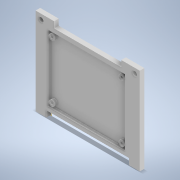
# Autodesk Inventor part: RelayTray
Saved by Autodesk Inventor 2022 (Build 260153000, 153)
## iProperties
Created: 2022-01-15
Part Number: RelayTray
Material: Generic
Document SubType Name: Modeling
Designer: siwat
Density: 1 g/cm^3
Appearance: Default
VLDS_Profile: Default Part
VLDS_TimeStamp: 2022-02-27
VLDS_FailCnt: 3
VLDS_AcceptCnt: 0
Author: siwat
Autodesk Inventor part; units mm, degrees
ref_plane "YZ Plane" through (0, 0, 0) normal (1, 0, 0) x (0, 1, 0)
ref_plane "XZ Plane" through (0, 0, 0) normal (0, 1, 0) x (-1, 0, 0)
ref_plane "XY Plane" through (0, 0, 0) normal (0, 0, 1) x (1, 0, 0)
ref_plane "Work Plane1" through (-62.4151, 1.9295, 0) normal (0, 0, 1) x (1, 0, 0)
sketch "Sketch1" plane through (-62.4151, 1.9295, 0) normal (0, 0, 1) x (1, 0, 0)
  line L0 (-5.0959, -1.798) -> (62.2123, -1.798)
  line L1 (62.2123, -1.798) -> (62.2123, 54.509)
  line L2 (62.2123, 54.509) -> (-5.0959, 54.509)
  line L3 (-5.0959, 54.509) -> (-5.0959, -1.798)
  circle A0 centre (-1.5532, 51.0932) radius 1.5
  circle A1 centre (58.9247, 51.1571) radius 1.5
  point P0 (62.4151, -1.9295)
  dimension "d1" = 3
  dimension "d6" = 3
  constraints: 8 end point, 2 centre point, 2 parallel, 1 horizontal, 1 perpendicular
  measures "d1" diameter of A0
  measures "d6" diameter of A1
extrude "Extrusion1" add sketch "Sketch1" along normal blind 3
sketch "Sketch3" plane through (-62.4151, 1.9295, 3) normal (0, 0, 1) x (1, 0, 0)
  line L0 (52.7586, 47.7976) -> (2.7586, 47.7976)
  line L1 (2.7586, 47.7976) -> (2.7586, 4.7976)
  line L2 (2.7586, 4.7976) -> (52.7586, 4.7976)
  line L3 (52.7586, 4.7976) -> (52.7586, 47.7976)
  circle A0 centre (5.2586, 7.7976) radius 1
  circle A1 centre (5.2586, 7.7976) radius 1.85
  circle A2 centre (50.2586, 7.7976) radius 1
  circle A3 centre (50.2586, 7.7976) radius 1.85
  circle A4 centre (50.2586, 44.7976) radius 1
  circle A5 centre (50.2586, 44.7976) radius 1.85
  circle A6 centre (5.2586, 44.7976) radius 1
  circle A7 centre (5.2586, 44.7976) radius 1.85
  point P0 (62.4151, -1.9295)
  dimension "d7" = 50
  dimension "d8" = 43
  dimension "d9" = 2
  dimension "d10" = 3.7
  dimension "d11" = 3
  dimension "d12" = 2.5
  dimension "d13" = 2
  dimension "d14" = 3.7
  dimension "d15" = 2
  dimension "d16" = 3.7
  dimension "d17" = 2
  dimension "d18" = 3.7
  dimension "d19" = 3
  dimension "d20" = 2.5
  dimension "d21" = 2.5
  dimension "d22" = 3
  dimension "d23" = 2.5
  dimension "d24" = 3
  constraints: 8 centre point, 8 end point, 4 coincident, 2 parallel, 1 horizontal, 1 perpendicular
  measures "d7" distance of L1.end L2.end
  measures "d8" distance of L2.end L0.start
  measures "d9" diameter of A0
  measures "d10" diameter of A1
  measures "d11" distance from line of A0.centre L2
  measures "d12" distance from line of L1 A0.centre
  measures "d13" diameter of A2
  measures "d14" diameter of A3
  measures "d15" diameter of A4
  measures "d16" diameter of A5
  measures "d17" diameter of A6
  measures "d18" diameter of A7
  measures "d19" distance from line of L0 A6.centre
  measures "d20" distance from line of L1 A6.centre
  measures "d21" distance from line of L3 A4.centre
  measures "d22" distance from line of L0 A4.centre
  measures "d23" distance from line of L3 A2.centre
  measures "d24" distance from line of A2.centre L2
extrude "Extrusion3" cut sketch "Sketch3" against normal blind 2
sketch "Sketch4" plane through (-62.4151, 1.9295, 1) normal (0, 0, 1) x (1, 0, 0)
  circle A0 centre (50.2586, 7.7976) radius 1 projected
  circle A1 centre (50.2586, 7.7976) radius 1
  circle A2 centre (50.2586, 44.7976) radius 1 projected
  circle A3 centre (50.2586, 44.7976) radius 1
  circle A4 centre (5.2586, 44.7976) radius 1 projected
  circle A5 centre (5.2586, 44.7976) radius 1
  circle A6 centre (5.2586, 7.7976) radius 1 projected
  circle A7 centre (5.2586, 7.7976) radius 1
  point P0 (62.4151, -1.9295)
  constraints: 4 centre point, 4 coincident
extrude "Extrusion4" cut sketch "Sketch4" against normal through all
sketch "Sketch5" plane through (-62.4151, 1.9295, 3) normal (0, 0, 1) x (1, 0, 0)
  line L0 (-5.0959, -1.798) -> (62.2123, -1.798) projected
  line L1 (55.2123, -1.798) -> (1.9041, -1.798)
  line L2 (1.9041, -1.798) -> (1.9041, 2.202)
  line L3 (1.9041, 2.202) -> (55.2123, 2.202)
  line L4 (55.2123, 2.202) -> (55.2123, -1.798)
  line L5 (62.2123, 54.509) -> (-5.0959, 54.509) projected
  line L6 (6.9041, 54.509) -> (50.2123, 54.509)
  line L7 (50.2123, 54.509) -> (50.2123, 50.509)
  line L8 (50.2123, 50.509) -> (6.9041, 50.509)
  line L9 (6.9041, 50.509) -> (6.9041, 54.509)
  line L10 (62.2123, -1.798) -> (62.2123, 54.509) projected
  line L11 (-5.0959, 54.509) -> (-5.0959, -1.798) projected
  point P0 (62.4151, -1.9295)
  point P1 (50.2123, 52.509)
  point P2 (6.9041, 52.509)
  point P3 (1.9041, 0.202)
  point P4 (55.2123, 0.202)
  dimension "d29" = 4
  dimension "d30" = 4
  dimension "d31" = 12
  dimension "d32" = 12
  dimension "d33" = 7
  dimension "d34" = 7
  constraints: 16 end point, 4 midpoint, 4 parallel, 2 horizontal, 2 perpendicular, 2 point on line
  measures "d29" distance between parallel lines of L0 L3
  measures "d30" distance between parallel lines of L5 L8
  measures "d31" distance from line of L10 point (50.212, 52.509)
  measures "d32" distance from line of L11 point (6.904, 52.509)
  measures "d33" distance from line of L11 point (1.904, 0.202)
  measures "d34" distance from line of L10 point (55.212, 0.202)
extrude "Extrusion5" cut sketch "Sketch5" against normal through all contours L2 L3 L4 L0 | L5 L7 L8 L9
body "Solid1"
